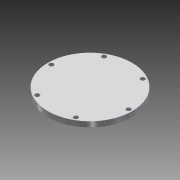
# Autodesk Inventor part: cap
Saved by Autodesk Inventor 2015 (Build 190159000, 159)
## iProperties
Created: 2015-02-28
Part Number: cap
Material: Generic
Document SubType Name: Modeling
Designer: Qiuyang
Density: 1 g/cm^3
Appearance: Default
Author: Qiuyang
Autodesk Inventor part; units mm, degrees
ref_plane "YZ Plane" through (0, 0, 0) normal (1, 0, 0) x (0, 1, 0)
ref_plane "XZ Plane" through (0, 0, 0) normal (0, 1, 0) x (-1, 0, 0)
ref_plane "XY Plane" through (0, 0, 0) normal (0, 0, 1) x (1, 0, 0)
sketch "Sketch4" plane through (0, 0, 0) normal (0, 1, 0) x (-1, 0, 0)
  circle A0 centre (0, 0) radius 50.8
  dimension "d2" = 101.6
  constraints: 1 centre point, 1 coincident
  measures "d2" diameter of A0
extrude "Extrusion3" add sketch "Sketch4" along normal blind 6.35
sketch "Sketch10" plane through (0, 6.35, 0) normal (0, 1, 0) x (1, 0, 0)
  circle A0 centre (-46.6725, 0) radius 2.667
  circle A1 centre (-23.3363, -40.4196) radius 2.667
  circle A2 centre (23.3362, -40.4196) radius 2.667
  circle A3 centre (46.6725, 0) radius 2.667
  circle A4 centre (23.3363, 40.4196) radius 2.667
  circle A5 centre (-23.3362, 40.4196) radius 2.667
  point P0 (0, 0)
  dimension "d41" = 5.334
  dimension "d44" = 360
  constraints: 6 centre point, 13 other
  measures "d41" diameter of A0
extrude "Extrusion6" cut sketch "Sketch10" against normal blind 6.35
body "Solid3"
